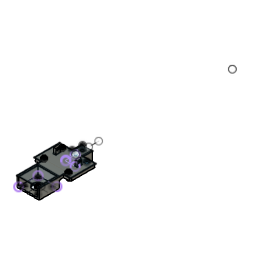
yCarriage (Autodesk Fusion 360 design; units mm, degrees)
Autodesk Fusion 360 part; units mm, degrees
sketch "Esquisse1" plane through (0, 0, 0) normal (0, 0, 1) x (1, 0, 0)
  line L0 (-40, -28) -> (-40, 28)
  line L1 (-40, 28) -> (-12, 28)
  line L2 (-12, 28) -> (-12, 49)
  line L3 (-12, 49) -> (12, 49)
  line L4 (12, 49) -> (12, 28)
  line L5 (12, 28) -> (40, 28)
  line L6 (40, 28) -> (40, -28)
  line L7 (40, -28) -> (24.5, -28)
  line L8 (24.5, -28) -> (24.5, -82)
  line L9 (24.5, -82) -> (-24.5, -82)
  line L10 (-24.5, -82) -> (-24.5, -28)
  line L11 (-24.5, -28) -> (-40, -28)
  circle A0 centre (-27.1, 21.1) radius 2.4
  circle A1 centre (-0.1034, 38.65) radius 2.9
  circle A2 centre (-27.1, -19.45) radius 2.4
  circle A3 centre (27.1, 21.1) radius 2.4
  circle A4 centre (27.1, -19.45) radius 2.4
  circle A5 centre (-0.0905, 23.6) radius 2.9
  line L12 (21.4, 11) -> (26.4, 11)
  line L13 (26.4, 11) -> (26.4, 1)
  line L14 (26.4, 1) -> (21.4, 1)
  line L15 (21.4, 1) -> (21.4, 11)
  line L16 (-21.4, 1) -> (-21.4, 11)
  line L17 (-26.4, 11) -> (-26.4, 1)
  line L18 (-26.4, 1) -> (-21.4, 1)
  line L19 (-21.4, 11) -> (-26.4, 11)
  line L20 (-24.5, -37) -> (24.5, -37)
  circle A6 centre (27.1, 21.1) radius 3.3
  circle A7 centre (27.1, -19.45) radius 3.3
  circle A8 centre (-27.1, 21.1) radius 3.3
  circle A9 centre (-27.1, -19.45) radius 3.3
  line L21 (10, 362.4031) -> (10, 362.403)
  line L22 (10, 49) -> (10, 28)
  line L23 (10, 28) -> (12, 28)
  line L24 (0, 75) -> (0, 52.7229) construction
  line L25 (-10, 49) -> (-10, 28)
  line L26 (-10, 28) -> (-12, 28)
  line L27 (21, -82) -> (21, -39)
  line L28 (21, -39) -> (-21, -39)
  line L29 (-21, -39) -> (-21, -82)
  line L30 (0, 1.75) -> (0, 22.5) construction
  line L31 (1.75, 0) -> (22.5, 0) construction
  dimension "d1" = 80
  dimension "d3" = 56
  dimension "d4" = 21
  dimension "d5" = 24
  dimension "d6" = 54
  dimension "d7" = 15.5
  dimension "d8" = 4.8
  dimension "d9" = 5.8
  dimension "d11" = 12.9
  dimension "d12" = 6.9
  dimension "d13" = 4.8
  dimension "d14" = 40.55
  dimension "d15" = 10.35
  dimension "d16" = 5.8
  dimension "d17" = 15.05
  dimension "d18" = 12.1034
  dimension "d19" = 54.2
  dimension "d20" = 5
  dimension "d21" = 10
  dimension "d22" = 13.6
  dimension "d23" = 17
  dimension "d24" = 45
  dimension "d27" = 6.6
  dimension "d28" = 12.9
  dimension "d29" = 6.9
  dimension "d30" = 6.6
  dimension "d31" = 6.6
  dimension "d32" = 6.6
  dimension "d33" = 2
  dimension "d34" = 2
  dimension "d35" = 3.5
  dimension "d36" = 3.5
  constraint vertical L0
  constraint perpendicular L0 L1
  constraint perpendicular L1 L2
  constraint perpendicular L2 L3
  constraint perpendicular L3 L4
  constraint perpendicular L4 L5
  constraint perpendicular L5 L6
  constraint perpendicular L6 L7
  constraint perpendicular L5 L8
  constraint perpendicular L8 L9
  constraint perpendicular L9 L10
  constraint perpendicular L0 L11
  constraint equal L0 L6
  constraint horizontal L12
  constraint vertical L13
  constraint horizontal L14
  constraint vertical L15
  constraint coincident L10 L20.start
  constraint coincident L8 L20.end
  constraint perpendicular L8 L20
  constraint concentric A3 A6
  constraint coincident A4.centre A7.centre
  constraint coincident A0.centre A8.centre
  constraint coincident A2.centre A9.centre
  constraint perpendicular L3 L21
  constraint coincident L3 L22.start
  constraint perpendicular L3 L22
  constraint vertical L24
  constraint symmetric L4.end L24 L1.end
  constraint symmetric L22.start L24 L25.start
  constraint symmetric L22.end L24 L25.end
  constraint coincident L9 L27.start
  constraint perpendicular L9 L27
  constraint perpendicular L27 L28
  constraint coincident L9 L29.end
  constraint perpendicular L9 L29
  constraint symmetric L2 L4 L30
  constraint symmetric L0 L6 L30
  constraint symmetric L8 L10 L30
  constraint symmetric L15 L16 L30
  constraint symmetric A2 A4 L30
  constraint symmetric L13 L17 L30
  constraint symmetric L14 L18 L30
  constraint symmetric L12 L19 L30
  constraint symmetric L22 L25 L30
  measures "d1" distance of L0 L6
  measures "d3" distance of L1 L11
  measures "d4" distance of L1.end L2.end
  measures "d5" distance of L2.end L3.end
  measures "d6" distance of L9.end L10.end
  measures "d7" distance of L0.start L10.end
  measures "d8" diameter of A0
  measures "d9" diameter of A1
  measures "d11" distance of L0 A0.centre
  measures "d12" distance of L1 A0.centre
  measures "d13" diameter of A2
  measures "d14" distance of A3.centre A4.centre
  measures "d15" distance of L3 A1.centre
  measures "d16" diameter of A5
  measures "d17" distance of A1.centre A5.centre
  measures "d18" distance of L4 A1.centre
  measures "d19" distance of A2.centre A4.centre
  measures "d20" distance of L12.start L12.end
  measures "d21" distance of L12.start L14.end
  measures "d22" distance of L6 L13
  measures "d23" distance of L5 L12
  measures "d24" distance of L9 L20
  measures "d27" diameter of A6
  measures "d28" distance of L6 A3.centre
  measures "d29" distance of L5 A3.centre
  measures "d30" diameter of A7
  measures "d31" diameter of A8
  measures "d32" diameter of A9
  measures "d33" distance of L4 L22
  measures "d34" distance of L20 L28
  measures "d35" distance of L8 L27
  measures "d36" distance of L10 L29
extrude "Extrusion1" add sketch "Esquisse1" against normal blind 23 contours L8 L9 L10 L20 L27 L28 L29 | L9 L27 L28 L29
extrude "Extrusion2" add sketch "Esquisse1" against normal blind 6.4 contours L0 L1 L3 L5 L6 L7 L8 L10 L11 L20 L22 L23 L25 L26 | L12 L13 L14 L15 | L16 L17 L18 L19
extrude "Extrusion3" add sketch "Esquisse1" against normal blind 14.14 contours A6
extrude "Extrusion4" add sketch "Esquisse1" against normal blind 14.14 contours A8
extrude "Extrusion5" add sketch "Esquisse1" against normal blind 14.14 contours A7
extrude "Extrusion6" add sketch "Esquisse1" against normal blind 14.14 contours A9
extrude "Extrusion7" add sketch "Esquisse1" against normal blind 26.4 contours L2 L3 L25 L26 | L3 L4 L22 L23
extrude "Extrusion8" cut sketch "Esquisse1" against normal blind 20 contours L9 L27 L28 L29
extrude "Extrusion9" add sketch "Esquisse1" along normal blind 12 contours L12 L13 L14 L15 | L16 L17 L18 L19
sketch "Esquisse2" plane through (26.4, 0, 0) normal (1, 0, 0) x (0, 1, 0)
  line L0 (1, 0) -> (11, 0)
  line L1 (11, 0) -> (11, 12)
  line L2 (11, 12) -> (1, 12)
  line L3 (1, 12) -> (1, 0)
  line L4 (8.84, 7.1) -> (3.16, 7.1)
  line L5 (3.16, 7.1) -> (3.16, 9.4)
  line L6 (3.16, 9.4) -> (8.84, 9.4)
  line L7 (8.84, 9.4) -> (8.84, 7.1)
  dimension "d53" = 2.6
  dimension "d54" = 2.3
  dimension "d55" = 2.16
  dimension "d56" = 2.16
  constraint horizontal L4
  constraint vertical L5
  constraint horizontal L6
  constraint vertical L7
  measures "d53" distance of L2 L6
  measures "d54" distance of L4 L6
  measures "d55" distance of L1 L7
  measures "d56" distance of L3 L5
extrude "Extrusion10" cut sketch "Esquisse2" against normal blind 90 contours L4 L5 L6 L7
sketch "Esquisse3" plane through (0, 0, 0) normal (0, 0, 1) x (1, 0, 0)
sketch "Esquisse4" plane through (0, 0, -20) normal (0, 0, 1) x (-1, 0, 0)
  line L0 (-21, 82) -> (-21, 39)
  line L1 (-21, 39) -> (21, 39)
  line L2 (21, 39) -> (21, 82)
  line L3 (21, 82) -> (-21, 82)
  circle A0 centre (15.6, 44.4) radius 1.5
  line L4 (21, 39) -> (21, 82) construction
  line L5 (-21, 39) -> (21, 39) construction
  circle A1 centre (-15.6, 44.4) radius 1.5
  circle A2 centre (15.6, 75.6) radius 1.5
  circle A3 centre (-15.6, 75.6) radius 1.5
  line L6 (21, 60.5) -> (-21, 60.5) construction
  line L7 (0, 39) -> (0, 82) construction
  circle A4 centre (0, 60.5) radius 11.05
  dimension "d59" = 3
  dimension "d60" = 5.4
  dimension "d61" = 5.4
  dimension "d64" = -31.2
  dimension "d65" = 31.2
  dimension "d66" = 22.1
  constraint midpoint L4 L6.start
  constraint midpoint L0 L6.end
  constraint midpoint L5 L7.start
  constraint midpoint L3 L7.end
  constraint midpoint L6 A4.centre
  measures "d59" diameter of A0
  measures "d60" distance of A0.centre L4
  measures "d61" distance of A0.centre L5
  measures "d66" diameter of A4
extrude "Extrusion11" cut sketch "Esquisse4" against normal blind 5 contours A0 | A1 | A2 | A3 | A4
fillet "Congé1" radius 2.5 1 edges at (40, -28, -3.2)
fillet "Congé2" radius 2.5 1 edges at (40, 28, -3.2)
fillet "Congé3" radius 2.5 1 edges at (-40, 28, -3.2)
fillet "Congé4" radius 2.5 1 edges at (-40, -28, -3.2)
fillet "Congé5" radius 0.8 1 edges at (-21.4, 6, 9.4)
fillet "Congé6" radius 0.8 1 edges at (26.4, 6, 9.4)
fillet "Congé7" radius 0.8 1 edges at (21.4, 6, 9.4)
fillet "Congé8" radius 0.8 1 edges at (-26.4, 6, 9.4)
fillet "Congé9" radius 2.5 1 edges at (0, -37, -6.4)
extrude "Extrusion12" add sketch "Esquisse4" along normal blind 0.5
chamfer "Chanfrein1" distance 0.8 angle 45 1 faces at (-23.8164, 20.7714, -8.98)
chamfer "Chanfrein2" distance 0.8 angle 45 1 faces at (-23.8164, -19.7786, -8.98)
chamfer "Chanfrein3" distance 0.8 angle 45 1 faces at (30.3836, 20.7714, -8.98)
chamfer "Chanfrein4" distance 0.8 angle 45 1 faces at (30.3836, -19.7786, -8.98)
